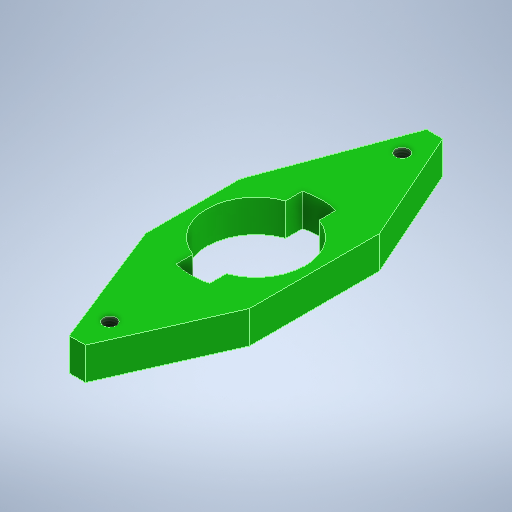
# Autodesk Inventor part: Axe centrale
Saved by Autodesk Inventor 2026.2 (Build 302298010, 298A)
## iProperties
Created: 2026-03-16
Part Number: Axe centrale
Material: Générique
Document SubType Name: Modeling
Designer: genon
Density: 1 g/cm^3
Appearance: Vert foncé
Author: genon
Autodesk Inventor part; units mm, degrees
ref_plane "YZ Plane" through (0, 0, 0) normal (1, 0, 0) x (0, 1, 0)
ref_plane "XZ Plane" through (0, 0, 0) normal (0, 1, 0) x (-1, 0, 0)
ref_plane "XY Plane" through (0, 0, 0) normal (0, 0, 1) x (1, 0, 0)
sketch "Esquisse1" plane through (0, 0, 0) normal (0, 1, 0) x (-1, 0, 0)
  circle A0 centre (0, 0) radius 15.15
  line L0 (0, 0) -> (18, 0)
  line L1 (18, 0) -> (18, -13.096)
  line L2 (18, 0) -> (18, 16)
  line L3 (0, 0) -> (-18, 0)
  line L4 (-18, 0) -> (-18, -20)
  line L5 (-18, 0) -> (-18, 20)
  line L6 (0, 0) -> (0, 55)
  line L7 (0, 0) -> (55, 0) construction
  line L8 (0, 55) -> (-2.5, 55)
  line L9 (-2.5, 55) -> (-18, 20)
  line L10 (0, 55) -> (2.5, 55)
  line L11 (2.5, 55) -> (18, 16)
  line L12 (0, 0) -> (0, -55)
  line L13 (0, 0) -> (55, 0) construction
  line L14 (0, -55) -> (2.5, -55)
  line L15 (2.5, -55) -> (18, -13.096)
  line L16 (0, -55) -> (-2.5, -55)
  line L17 (-2.5, -55) -> (-18, -20)
  line L18 (0, 0) -> (5.15, 0)
  line L19 (5.15, 0) -> (5.15, -19.4422)
  line L20 (0, 0) -> (-5.15, 0)
  line L21 (-5.15, 0) -> (-5.15, -19.4422)
  line L22 (-5.15, 0) -> (-5.15, 19.4422)
  line L23 (5.15, 0) -> (5.15, 19.4422)
  arc A1 (-5.15, -19.4422) -> (5.15, -19.4422) centre (0, 0.1906) ccw
  arc A2 (5.15, 19.4422) -> (-5.15, 19.4422) centre (0, 0.0132) ccw
  point P0 (5.15, -14.2478)
  point P1 (-5.1, -19.4422)
  point P2 (-5.15, -14.2478)
  point P3 (-5.15, 14.2478)
  point P4 (5.15, 14.2478)
  dimension "d0" = 30.3
  dimension "d1" = 18
  dimension "d3" = 90
  dimension "d4" = 16
  dimension "d6" = 18
  dimension "d7" = 20
  dimension "d8" = 20
  dimension "d9" = 55
  dimension "d10" = 90
  dimension "d11" = 2.5
  dimension "d12" = 2.5
  dimension "d13" = 55
  dimension "d14" = 90
  dimension "d15" = 2.5
  dimension "d16" = 90
  dimension "d17" = 2.5
  dimension "d19" = 5.15
  dimension "d20" = 5.15
  dimension "d34" = 10.3
  dimension "d35" = 29.397
  constraints: 48 end point, 9 perpendicular, 5 horizontal, 5 point on line, 4 point on circle, 3 centre point, 3 vertical, 2 coincident
  measures "d0" diameter of A0
  measures "d1" distance of L0.start L0.end
  measures "d3" angle of L0 L1
  measures "d4" distance of L0.end L2.end
  measures "d6" distance of L0.start L3.end
  measures "d7" distance of L3.end L4.end
  measures "d8" distance of L3.end L5.end
  measures "d9" distance of L0.start L6.end
  measures "d10" angle of L7 L6
  measures "d11" distance of L6.end L8.end
  measures "d12" distance of L6.end L10.end
  measures "d13" distance of L0.start L12.end
  measures "d14" angle of L12 L13
  measures "d15" distance of L12.end L14.end
  measures "d16" angle of L14 L12
  measures "d17" distance of L12.end L16.end
  measures "d19" distance of L18.start L18.end
  measures "d20" distance of L18.start L20.end
  measures "d34" distance of A1.start L19.end
extrude "Extrusion1" add sketch "Esquisse1" along normal blind 10 contours L0 L1 L15 L14 L12 A1 L19 A0 | A0 L23 A2 L6 L10 L11 L2 L0 | A0 L3 L5 L9 L8 L6 A2 L22 | L21 A1 L12 L16 L17 L4 L3 A0
sketch "Esquisse2" plane through (0, 10, 0) normal (0, 1, 0) x (1, 0, 0)
  line L0 (-2.5, -55) -> (2.5, -55) projected
  line L1 (0, -55) -> (0, -25)
  line L2 (0, -25) -> (-14.4231, -25)
  line L3 (-18, -16) -> (-2.5, -55) projected
  line L4 (0, -25) -> (15.7857, -25)
  line L5 (2.5, -55) -> (18, -20) projected
  line L6 (0, -55) -> (0, -45)
  line L7 (0, -45) -> (0, -35)
  line L8 (0, 0) -> (-7.091, 0)
  point P0 (0, 45)
  dimension "d23" = 30
  dimension "d24" = 10
  dimension "d25" = 10
  constraints: 12 end point, 4 point on line, 2 horizontal, 1 coincident, 1 midpoint, 1 perpendicular, 1 symmetric about line, 1 vertical
  measures "d23" distance of L1.start L1.end
  measures "d24" distance of L1.start L6.end
  measures "d25" distance of L6.end L7.end
hole "Perçage1" at (0, 10, 45) at (0, 10, -45) direction (0, -1, 0) diameter 4.134 end through all thread size "M5x0.8" class "6H" standard "ISO Metric profile"
